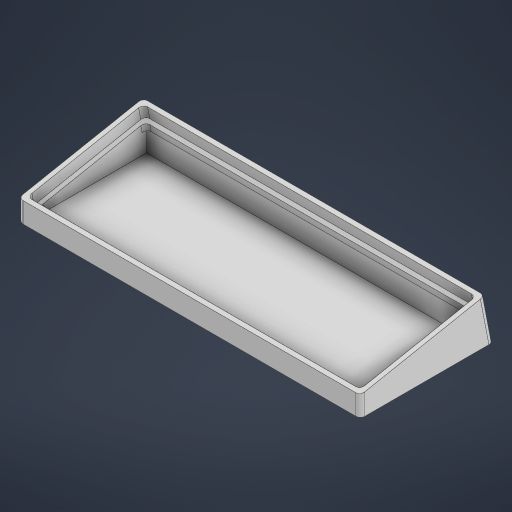
# Autodesk Inventor part: housing
Saved by Autodesk Inventor 2024.2 (Build 282272000, 272)
## iProperties
Created: 2024-12-04
Part Number: housing
Material: Generic
Document SubType Name: Modeling
Designer: Moe
Density: 1 g/cm^3
Appearance: Default
Author: Moe
Autodesk Inventor part; units mm, degrees
ref_plane "YZ Plane" through (0, 0, 0) normal (1, 0, 0) x (0, 1, 0)
ref_plane "XZ Plane" through (0, 0, 0) normal (0, 1, 0) x (-1, 0, 0)
ref_plane "XY Plane" through (0, 0, 0) normal (0, 0, 1) x (1, 0, 0)
sketch "Sketch1" plane through (0, 0, 0) normal (1, 0, 0) x (0, 1, 0)
  line L0 (0, 0) -> (9, 0)
  line L1 (9, 0) -> (19.6853, -54.9711)
  line L2 (9, 0) -> (65, 0) construction
  line L3 (19.6853, -54.9711) -> (0, -58.7976)
  line L4 (19.6853, -54.9711) -> (39.7391, -54.9711) construction
  line L5 (0, -58.7976) -> (0, 0)
  dimension "d0" = 9
  dimension "d1" = 56
  dimension "d2" = 79
  dimension "d5" = 169
  constraints: 12 end point, 3 horizontal, 2 equal length, 1 vertical
  measures "d0" distance of L0.start L0.end
  measures "d1" distance of L0.end L1.end
  measures "d2" angle of L1 L2
  measures "d5" angle of L3 L4
extrude "Extrusion1" add sketch "Sketch1" along normal blind 151
fillet "Fillet1" radius 2 4 edges at (151, 9.8427, -56.8843) (151, 4.5, 0) (0, 9.8427, -56.8843) (0, 4.5, 0)
sketch "Sketch2" plane through (2, 9, 0) normal (0, 0.9816272, 0.190809) x (1, 0, 0)
  ellipse E0 centre (0, 2.0374) end of major axis (0, 0) minor radius 2 (-2, 2.0374) -> (0, 0) ccw projected
  line L0 (0, 0) -> (147, 0) projected
  ellipse E1 centre (147, 2.0374) end of major axis (147, 0) minor radius 2 (147, 0) -> (149, 2.0374) ccw projected
  line L1 (149, 54) -> (149, 2.0374) projected
  arc A0 (149, 54) -> (147, 56) centre (147, 54) ccw projected
  line L2 (0, 56) -> (147, 56) projected
  arc A1 (0, 56) -> (-2, 54) centre (0, 54) ccw projected
  line L3 (-2, 54) -> (-2, 2.0374) projected
  line L4 (2, 54) -> (145, 54)
  line L5 (147, 52) -> (147, 4)
  line L6 (145, 2) -> (2, 2)
  line L7 (0, 4) -> (0, 52)
  arc A2 (2, 54) -> (0, 52) centre (2, 52) ccw
  arc A3 (0, 4) -> (2, 2) centre (2, 4) ccw
  arc A4 (145, 2) -> (147, 4) centre (145, 4) ccw
  arc A5 (147, 52) -> (145, 54) centre (145, 52) ccw
  point P0 (-2, -1.7173)
  dimension "d7" = 2
  dimension "d8" = 2
  dimension "d9" = 2
  dimension "d10" = 2
  dimension "d11" = 2
  constraints: 8 end point, 8 point on circle, 8 tangent, 4 centre point, 3 equal radius, 2 parallel, 1 horizontal, 1 perpendicular, 2 other
  measures "d7" distance between parallel lines of L2 L4
  measures "d8" distance between parallel lines of L3 L7
  measures "d9" distance between parallel lines of L0 L6
  measures "d10" distance between parallel lines of L1 L5
  measures "d11" radius of A2
extrude "Extrusion2" cut sketch "Sketch2" against normal blind 5 contours L4 A5 L5 A4 L6 A3 L7 A2
sketch "Sketch3" plane through (2, 4.0919, -0.954) normal (0, 0.9816272, 0.190809) x (1, 0, 0)
  line L0 (4, 52) -> (143, 52)
  line L1 (145, 50) -> (145, 6)
  line L2 (143, 4) -> (4, 4)
  line L3 (2, 6) -> (2, 50)
  line L4 (2, 54) -> (145, 54) projected
  line L5 (147, 52) -> (147, 4) projected
  line L6 (145, 2) -> (2, 2) projected
  line L7 (0, 4) -> (0, 52) projected
  arc A0 (4, 52) -> (2, 50) centre (4, 50) ccw
  arc A1 (2, 6) -> (4, 4) centre (4, 6) ccw
  arc A2 (143, 4) -> (145, 6) centre (143, 6) ccw
  arc A3 (145, 50) -> (143, 52) centre (143, 50) ccw
  point P0 (-2, -1.7173)
  dimension "d14" = 2
  dimension "d15" = 2
  dimension "d16" = 2
  dimension "d17" = 2
  dimension "d18" = 2
  constraints: 8 end point, 8 point on circle, 8 tangent, 4 centre point, 3 equal radius, 2 parallel, 1 horizontal, 1 perpendicular
  measures "d14" distance between parallel lines of L4 L0
  measures "d15" distance between parallel lines of L5 L1
  measures "d16" distance between parallel lines of L6 L2
  measures "d17" distance between parallel lines of L7 L3
  measures "d18" radius of A0
extrude "Extrusion3" cut sketch "Sketch3" against normal blind 3
ref_plane "Work Plane1" through (75.5, 0, 0) normal (1, 0, 0) x (0, 0, -1)
sketch "Sketch4" plane through (75.5, 0, 0) normal (1, 0, 0) x (0, 0, -1)
  line L0 (4.8806, 4.8551) -> (5.453, 1.9102) projected
  line L1 (50.6078, 10.6874) -> (7.4162, 2.2918) projected
  line L2 (51.9987, 14.0139) -> (52.5711, 11.0691) projected
  line L3 (5.453, 1.9102) -> (52.5711, 11.0691)
  line L4 (5.453, 1.9102) -> (7.4162, 2.2918) projected
  line L5 (5.453, 1.9102) -> (52.5711, 1.9102)
  line L6 (52.5711, 1.9102) -> (52.5711, 11.0691)
  line L7 (5.453, 1.9102) -> (52.5711, 11.0691)
  point P0 (0, 0)
  point P1 (7.4162, 2.2918)
  constraints: 8 end point, 1 collinear, 1 horizontal, 1 perpendicular
extrude "Extrusion4" cut sketch "Sketch4" along normal mid plane 143
body "Solid1"
